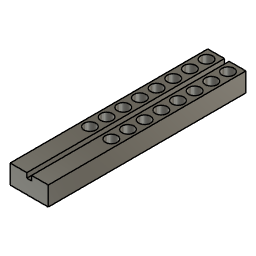
tree_template (Autodesk Fusion 360 design; units mm, degrees)
Autodesk Fusion 360 part; units mm, degrees
sketch "tree" plane through (0, 0, 0) normal (0, 0, 1) x (1, 0, 0)
  line L0 (0, 0) -> (0, 94.3715) construction
  circle A0 centre (-4.5, 30) radius 2.5
  circle A1 centre (4.5, 30) radius 2.5
  circle A2 centre (-4.5, 37) radius 2.5
  circle A3 centre (4.5, 37) radius 2.5
  circle A4 centre (-4.5, 44) radius 2.5
  circle A5 centre (4.5, 44) radius 2.5
  circle A6 centre (-4.5, 51) radius 2.5
  circle A7 centre (4.5, 51) radius 2.5
  circle A8 centre (-4.5, 58) radius 2.5
  circle A9 centre (4.5, 58) radius 2.5
  circle A10 centre (-4.5, 65) radius 2.5
  circle A11 centre (4.5, 65) radius 2.5
  circle A12 centre (-4.5, 72) radius 2.5
  circle A13 centre (4.5, 72) radius 2.5
  circle A14 centre (-4.5, 79) radius 2.5
  circle A15 centre (4.5, 79) radius 2.5
  line L1 (-1, 83) -> (1, 83)
  line L2 (1, 83) -> (1, 0)
  line L3 (1, 0) -> (-1, 0)
  line L4 (-1, 0) -> (-1, 83)
  dimension "d7" = 5
  dimension "d10" = 9
  dimension "d11" = 7
  dimension "d12" = 2
  dimension "d13" = 30
  dimension "d14" = 4
  constraint coincident L0.start origin
  constraint vertical L0
  constraint symmetric L0 A0.centre A1.centre
  constraint horizontal L1
  constraint vertical L2
  constraint horizontal L3
  constraint vertical L4
  constraint midpoint L0.start L3
  measures "d7" diameter of A0
  measures "d12" distance of L1.start L1.end
  measures "d13" distance of A0.centre L3
  measures "d14" distance of A14.centre L1
sketch "plate" plane through (0, 0, 0) normal (0, 0, 1) x (1, 0, 0)
  line L0 (-8, 83) -> (8, 83)
  line L1 (8, 83) -> (8, 0)
  line L2 (8, 0) -> (-8, 0)
  line L3 (-8, 0) -> (-8, 83)
  line L4 (0, 0) -> (0, 94.3715)
  point P0 (1, 83)
  dimension "d16" = 8
  constraint horizontal L0
  constraint vertical L1
  constraint horizontal L2
  constraint vertical L3
  constraint symmetric L1 L3 L4
  constraint coincident L0 P0
  constraint coincident L2 L4.start
  measures "d16" distance of L3 L4
extrude "Extrude1" add sketch "plate" against normal blind 8
extrude "Extrude2" cut sketch "tree" against normal through all contours A0 | A1 | A2 | A3 | A4 | A5 | A6 | A7 | A8 | A9 | A10 | A11 | A12 | A13 | A14 | A15
extrude "Extrude3" cut sketch "tree" against normal blind 2 contours L1 L2 L3 L4
equation "led_dia = 5 mm"
equation "wire_dia = 2 mm"
equation "led_vspace = 2 mm" comment "Vertical spacing between leds"
equation "led_hspace = 2 mm" comment "horizontal spacing between led and centerline of wire"
equation "wire_bottom_stickout = 30 mm" comment "How far the wire should expand beneath the center of the topmost led"
equation "wire_top_stickout = 4 mm" comment "How far the wire should extend above the center of the topmost led"
equation "d7 = led_dia"
equation "d10 = led_dia + led_hspace + wire_dia"
equation "d11 = led_dia + led_vspace"
equation "d12 = wire_dia"
equation "d13 = wire_bottom_stickout"
equation "d14 = wire_top_stickout"
equation "d16 = led_dia + led_hspace + 1 mm"
named bodies: "tree_template"
